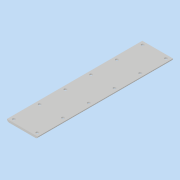
# Autodesk Inventor part: MidshipsSideGeneric
Saved by Autodesk Inventor 2017 (Build 210142000, 142)
## iProperties
Created: 2017-02-01
Part Number: MidshipsSideGeneric
Material: Generic
Document SubType Name: Modeling
Designer: techn
Density: 1 g/cm^3
Appearance: Default
Author: techn
Autodesk Inventor part; units mm, degrees
ref_plane "YZ Plane" through (0, 0, 0) normal (1, 0, 0) x (0, 1, 0)
ref_plane "XZ Plane" through (0, 0, 0) normal (0, 1, 0) x (-1, 0, 0)
ref_plane "XY Plane" through (0, 0, 0) normal (0, 0, 1) x (1, 0, 0)
sketch "Sketch3" plane through (0, 0, 0) normal (0, 1, 0) x (-1, 0, 0)
  line L0 (0, 0) -> (31.75, 0)
  line L1 (31.75, 0) -> (31.75, -139.7)
  line L2 (31.75, -139.7) -> (0, -139.7)
  line L3 (0, -139.7) -> (0, 0)
  dimension "d4" = 31.75
  dimension "d5" = 139.7
  constraints: 8 end point, 2 parallel, 1 horizontal, 1 perpendicular
  measures "d4" distance of L1.end L2.end
  measures "d5" distance of L0.end L1.end
extrude "Extrusion2" add sketch "Sketch3" along normal blind 2.286
sketch "Sketch5" plane through (0, 0, 0) normal (0, -1, 0) x (1, 0, 0)
  line L0 (0, -139.7) -> (0, 0) projected
  line L1 (0, 0) -> (-31.75, 0) projected
  circle A0 centre (-3.81, -3.429) radius 1.397
  dimension "d8" = 2.794
  dimension "d9" = 3.81
  dimension "d10" = 3.429
  constraints: 1 centre point
  measures "d8" diameter of A0
  measures "d9" distance from line of A0.centre L0
  measures "d10" distance from line of A0.centre L1
extrude "Extrusion3" cut sketch "Sketch5" against normal blind 2.286
chamfer "Chamfer1" distance 1.143 angle 45 1 edges at (-5.207, 0, -3.429)
pattern_linear "Rectangular Pattern1" count 6 spacing 26.5684 along (0, 0, -1) count 2 spacing 24.13 along (-1, 0, 0) of "Extrusion3", "Chamfer1"
fillet "Fillet1" radius 2.286 2 edges at (-31.75, 0, -69.85) (0, 0, -69.85)
body "Solid2"
